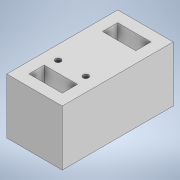
# Autodesk Inventor part: Wrist Base
Saved by Autodesk Inventor 2022 (Build 260153000, 153)
## iProperties
Created: 2022-03-10
Part Number: Wrist Base
Material: Generic
Document SubType Name: Modeling
Designer: shubh
Density: 1 g/cm^3
Appearance: Default
Author: shubh
Autodesk Inventor part; units mm, degrees
ref_plane "YZ Plane" through (0, 0, 0) normal (1, 0, 0) x (0, 1, 0)
ref_plane "XZ Plane" through (0, 0, 0) normal (0, 1, 0) x (-1, 0, 0)
ref_plane "XY Plane" through (0, 0, 0) normal (0, 0, 1) x (1, 0, 0)
sketch "Sketch1" plane through (0, 0, 0) normal (0, 1, 0) x (-1, 0, 0)
  line L0 (0, 0) -> (-12.7, 0)
  line L1 (-12.7, 0) -> (-12.7, -25.4)
  line L2 (-12.7, -25.4) -> (0, -25.4)
  line L3 (0, -25.4) -> (0, 0)
  line L4 (-2.54, -2.54) -> (-10.16, -2.54)
  line L5 (-10.16, -2.54) -> (-10.16, -6.0325)
  line L6 (-10.16, -6.0325) -> (-2.54, -6.0325)
  line L7 (-2.54, -6.0325) -> (-2.54, -2.54)
  circle A0 centre (-3.175, -8.5725) radius 0.635
  circle A1 centre (-9.525, -8.5725) radius 0.635
  line L8 (-2.54, -19.3675) -> (-10.16, -19.3675)
  line L9 (-10.16, -19.3675) -> (-10.16, -22.86)
  line L10 (-10.16, -22.86) -> (-2.54, -22.86)
  line L11 (-2.54, -22.86) -> (-2.54, -19.3675)
  dimension "d0" = 12.7
  dimension "d1" = 25.4
  dimension "d2" = 2.54
  dimension "d3" = 2.54
  dimension "d4" = 2.54
  dimension "d5" = 1.27
  dimension "d6" = 2.54
  dimension "d7" = 2.54
  dimension "d8" = 2.54
  constraints: 24 end point, 6 parallel, 3 horizontal, 3 perpendicular, 2 centre point, 2 equal length, 1 equal radius
  measures "d0" distance of L2.end L1.end
  measures "d1" distance of L1.end L0.end
  measures "d2" distance between parallel lines of L0 L4
  measures "d3" distance between parallel lines of L3 L7
  measures "d4" distance between parallel lines of L1 L5
  measures "d5" diameter of A0
  measures "d6" distance from line of L6 A0.centre
  measures "d7" distance from line of L6 A1.centre
  measures "d8" distance between parallel lines of L2 L10
extrude "Extrusion1" add sketch "Sketch1" along normal blind 12.7
extrude "Extrusion2" add sketch "Sketch1" along normal blind 0.508 contours L7 L6 L5 L4 | A0 | A1 | L11 L10 L9 L8
body "Solid1"
